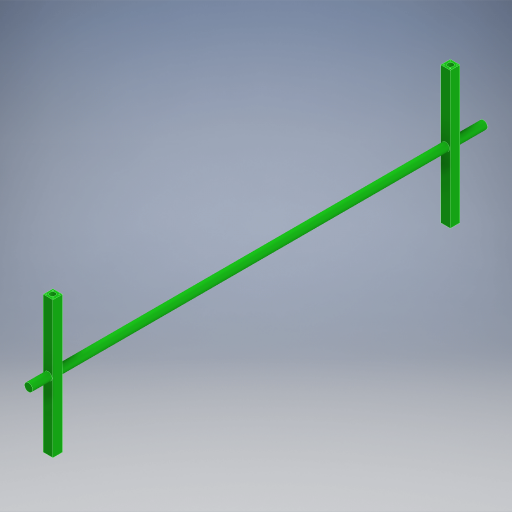
# Autodesk Inventor part: Soporte Superior bandeja
Saved by Autodesk Inventor 2024.3 (Build 283343010, 343A)
## iProperties
Created: 2025-05-04
Part Number: Soporte Superior bandeja
Material: Steel, Mild
Document SubType Name: Modeling
Designer: Gary
Density: 7.85 g/cm^3
Appearance: Dark Green
Author: Gary
Autodesk Inventor part; units mm, degrees
ref_plane "YZ Plane" through (0, 0, 0) normal (1, 0, 0) x (0, 1, 0)
ref_plane "XZ Plane" through (0, 0, 0) normal (0, 1, 0) x (-1, 0, 0)
sketch "Sketch1" plane through (0, 0, 0) normal (0, 0, 1) x (1, 0, 0)
  line L0 (0, 0) -> (-120, 0)
  line L1 (-120, 0) -> (-120, -1650)
  line L2 (-120, -1650) -> (0, -1650)
  line L3 (0, -1650) -> (0, 0)
  dimension "d0" = 120
  dimension "d1" = 1650
  constraints: 8 end point, 2 parallel, 1 horizontal, 1 perpendicular
  measures "d0" distance of L2.end L1.end
  measures "d1" distance of L1.end L0.end
extrude "Extrusion1" add sketch "Sketch1" along normal blind 120
sketch "Sketch2" plane through (0, 0, 120) normal (0, 0, 1) x (1, 0, 0)
  circle A0 centre (-60, -825) radius 50
  line L0 (-120, -1650) -> (0, -1650) projected
  line L1 (-120, 0) -> (-120, -1650) projected
  point P0 (0, 0)
  point P1 (-60, -1650)
  point P2 (-120, -825)
  dimension "d4" = 100
  dimension "d6" = 825
  dimension "d8" = 60
  constraints: 2 midpoint, 1 centre point
  measures "d4" diameter of A0
  measures "d6" distance from line of A0.centre L0
  measures "d8" distance of point (-120, -825) A0.centre
extrude "Extrusion2" add sketch "Sketch2" along normal blind 4860
sketch "Sketch11" plane through (0, 0, 0) normal (0, 0, -1) x (-1, 0, 0)
  circle A0 centre (60, -825) radius 50 projected
  circle A1 centre (60, -825) radius 50
  point P0 (0, 0)
  dimension "d52" = 100
  constraints: 1 centre point, 1 coincident
  measures "d52" diameter of A1
extrude "Extrusion6" add sketch "Sketch11" along normal blind 130
sketch "Sketch12" plane through (-60, -825, -130) normal (0, 0, -1) x (-1, 0, 0)
  circle A0 centre (0, 0) radius 50
  point P0 (-60, 825)
  dimension "d48" = 100
  dimension "d49" = 827.1789
  constraints: 1 centre point
  measures "d48" diameter of A0
  measures "d49" distance of A0.centre point (-60, 825)
extrude "Extrusion7" add sketch "Sketch12" along normal blind 115
sketch "Sketch13" plane through (-120, 0, 0) normal (0, 1, 0) x (1, 0, 0)
  line L0 (120, 0) -> (120, -120) projected
  line L1 (120, -120) -> (0, -120) projected
  line L2 (120, 0) -> (0, 0)
  line L3 (0, 0) -> (0, -120)
  line L4 (0, -120) -> (120, -120)
  line L5 (120, -120) -> (120, 0)
  constraints: 8 end point, 2 parallel, 1 horizontal, 1 perpendicular
extrude "Extrusion8" add sketch "Sketch13" along normal blind 32
sketch "Sketch14" plane through (-120, 32, 0) normal (0, 1, 0) x (1, 0, 0)
  circle A0 centre (20, -100) radius 5.5
  circle A1 centre (20, -20) radius 5.5
  circle A2 centre (100, -100) radius 5.5
  circle A3 centre (100, -20) radius 5.5
  circle A4 centre (60, -60) radius 35
  line L0 (0, 0) -> (0, -120) projected
  line L1 (0, -120) -> (120, -120) projected
  line L2 (120, 0) -> (0, 0) projected
  line L3 (120, -120) -> (120, 0) projected
  dimension "d59" = 20
  dimension "d60" = 20
  dimension "d61" = 20
  dimension "d62" = 11
  dimension "d63" = 11
  dimension "d64" = 11
  dimension "d65" = 11
  dimension "d66" = 20
  dimension "d67" = 20
  dimension "d68" = 20
  dimension "d69" = 20
  dimension "d70" = 20
  dimension "d71" = 70
  dimension "d72" = 60
  dimension "d73" = 60
  constraints: 5 centre point
  measures "d59" distance from line of L0 A0.centre
  measures "d60" distance from line of L1 A0.centre
  measures "d61" distance from line of L2 A1.centre
  measures "d62" diameter of A0
  measures "d63" diameter of A1
  measures "d64" diameter of A2
  measures "d65" diameter of A3
  measures "d66" distance from line of L0 A1.centre
  measures "d67" distance from line of L1 A2.centre
  measures "d68" distance from line of L3 A2.centre
  measures "d69" distance from line of L2 A3.centre
  measures "d70" distance from line of L3 A3.centre
  measures "d71" diameter of A4
  measures "d72" distance from line of L0 A4.centre
  measures "d73" distance from line of L1 A4.centre
extrude "Extrusion9" cut sketch "Sketch14" against normal blind 100 contours A0 | A1 | A2 | A3
extrude "Extrusion10" cut sketch "Sketch14" against normal blind 100 contours A4
sketch "Sketch15" plane through (-60, -825, 4980) normal (0, 0, 1) x (1, 0, 0)
  line L0 (60, 857) -> (60, -857) projected
  line L1 (-60, -857) -> (60, -857)
  line L2 (60, -857) -> (60, 857)
  line L3 (60, 857) -> (-60, 857)
  line L4 (-60, 857) -> (-60, -857)
  line L5 (-60, -857) -> (60, 857) construction
  line L6 (60, -857) -> (-60, 857) construction
  point P0 (60, 825)
  point P1 (0, 0)
  dimension "d79" = 4.005
  dimension "d80" = 120
  constraints: 12 end point, 2 midpoint, 2 parallel, 1 horizontal, 1 perpendicular
  measures "d79" angle of L5 L0
  measures "d80" distance between parallel lines of L0 L4
extrude "Extrusion11" add sketch "Sketch15" along normal blind 120
sketch "Sketch16" plane through (-120, 32, 4980) normal (0, 1, 0) x (1, 0, 0)
  circle A0 centre (20, -100) radius 5.5
  circle A1 centre (20, -20) radius 5.5
  circle A2 centre (100, -100) radius 5.5
  circle A3 centre (100, -20) radius 5.5
  circle A4 centre (54.487, -60) radius 35
  line L0 (0, 0) -> (0, -120) projected
  line L1 (120, -120) -> (0, -120) projected
  line L2 (120, 0) -> (0, 0) projected
  line L3 (120, 0) -> (120, -120) projected
  point P0 (120, 4980)
  dimension "d83" = 11
  dimension "d84" = 11
  dimension "d85" = 11
  dimension "d86" = 11
  dimension "d87" = 20
  dimension "d88" = 20
  dimension "d89" = 20
  dimension "d90" = 20
  dimension "d91" = 20
  dimension "d92" = 20
  dimension "d93" = 20
  dimension "d94" = 20
  dimension "d95" = 60
  dimension "d96" = 70
  dimension "d97" = 65.513
  constraints: 5 centre point
  measures "d83" diameter of A0
  measures "d84" diameter of A1
  measures "d85" diameter of A2
  measures "d86" diameter of A3
  measures "d87" distance from line of L0 A0.centre
  measures "d88" distance from line of L1 A0.centre
  measures "d89" distance from line of L2 A1.centre
  measures "d90" distance from line of L0 A1.centre
  measures "d91" distance from line of L1 A2.centre
  measures "d92" distance from line of L3 A2.centre
  measures "d93" distance from line of L2 A3.centre
  measures "d94" distance from line of L3 A3.centre
  measures "d95" distance from line of L2 A4.centre
  measures "d96" diameter of A4
  measures "d97" distance from line of A4.centre L3
extrude "Extrusion12" cut sketch "Sketch16" against normal blind 100 contours A0 | A1 | A2 | A3
extrude "Extrusion13" cut sketch "Sketch16" against normal blind 100 contours A4
sketch "Sketch17" plane through (-60, -825, 5100) normal (0, 0, 1) x (1, 0, 0)
  circle A0 centre (0, 0) radius 50
  point P0 (60, 825)
  dimension "d102" = 100
  dimension "d103" = 827.1789
  constraints: 1 centre point
  measures "d102" diameter of A0
  measures "d103" distance of point (60, 825) A0.centre
extrude "Extrusion14" add sketch "Sketch17" along normal blind 130
sketch "Sketch18" plane through (-60, -825, 5230) normal (0, 0, 1) x (1, 0, 0)
  circle A0 centre (0, 0) radius 50
  point P0 (60, 825)
  dimension "d106" = 100
  dimension "d107" = 827.1789
  constraints: 1 centre point
  measures "d106" diameter of A0
  measures "d107" distance of point (60, 825) A0.centre
extrude "Extrusion15" add sketch "Sketch18" along normal blind 115
sketch "Sketch20" plane through (-60, -825, -245) normal (0, 0, -1) x (-1, 0, 0)
  circle A0 centre (0, 0) radius 50
  point P0 (-60, 825)
  dimension "d113" = 100
  dimension "d114" = 827.1789
  constraints: 1 centre point
  measures "d113" diameter of A0
  measures "d114" distance of A0.centre point (-60, 825)
extrude "Extrusion16" add sketch "Sketch20" along normal blind 50
sketch "Sketch21" plane through (-120, -1650, 0) normal (0, -1, 0) x (1, 0, 0)
  line L0 (0, 0) -> (0, 120) projected
  line L1 (0, 120) -> (120, 120)
  line L2 (120, 120) -> (120, 0)
  line L3 (120, 0) -> (0, 0)
  line L4 (0, 0) -> (0, 120)
  constraints: 8 end point, 2 parallel, 1 horizontal, 1 perpendicular
extrude "Extrusion17" add sketch "Sketch21" along normal blind 32
ref_plane "Work Plane6" through (-120, -825, 0) normal (0, 1, 0) x (1, 0, 0)
mirror "Mirror7" about plane through (-120, -825, 0) normal (0, 1, 0) of "Extrusion10", "Extrusion9"
mirror "Mirror8" about plane through (-120, -825, 0) normal (0, 1, 0) of "Extrusion13", "Extrusion12"
sketch "Sketch22" plane through (-60, -825, -295) normal (0, 0, -1) x (-1, 0, 0)
  circle A0 centre (0, 0) radius 50 projected
  circle A1 centre (0, 0) radius 50
  point P0 (-60, 825)
  constraints: 1 centre point, 1 coincident
extrude "Extrusion18" add sketch "Sketch22" along normal blind 60
body "Solid1"
